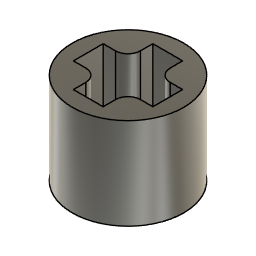
ring (Autodesk Fusion 360 design; units mm, degrees)
Autodesk Fusion 360 part; units mm, degrees
sketch "Sketch1" plane through (0, 0, 0) normal (0, 0, 1) x (1, 0, 0)
  line L0 (-6.1203, 21.0064) -> (-1.3403, 21.0064)
  line L1 (-1.3403, 21.0064) -> (-1.3403, 19.2164)
  line L2 (-1.3403, 19.2164) -> (-6.1203, 19.2164)
  line L3 (-6.1203, 19.2164) -> (-6.1203, 21.0064)
  line L4 (-6.1203, 19.2164) -> (-4.6253, 19.2164)
  line L5 (-4.6253, 19.2164) -> (-2.8353, 19.2164)
  line L6 (-4.6253, 19.2164) -> (-4.6253, 17.7214)
  line L7 (-4.6253, 17.7214) -> (-2.8353, 17.7214)
  line L8 (-2.8353, 17.7214) -> (-2.8353, 17.8)
  line L9 (-2.8353, 17.8) -> (-2.8353, 19.2164)
  line L10 (-4.6253, 19.2164) -> (-4.6253, 21.0064)
  line L11 (-2.8353, 19.2164) -> (-2.8353, 21.0064)
  line L12 (-2.8353, 21.0064) -> (-4.6253, 21.0064)
  line L13 (-4.6253, 21.0064) -> (-4.6253, 22.5014)
  line L14 (-4.6253, 22.5014) -> (-2.8353, 22.5014)
  line L15 (-2.8353, 22.5014) -> (-2.8353, 21.0064)
  circle A0 centre (-5.3728, 18.4689) radius 0.7475
  circle A1 centre (-2.0878, 18.4689) radius 0.7475
  circle A2 centre (-2.0878, 21.7539) radius 0.7475
  circle A3 centre (-5.3728, 21.7539) radius 0.7475
  circle A4 centre (-3.7303, 20.1114) radius 3.35
  dimension "d2" = 4.78
  dimension "d3" = 1.79
  dimension "d4" = 4.78
  dimension "d5" = 1.495
  dimension "d6" = 1.79
  dimension "d7" = 1.495
  dimension "d8" = 1.79
  dimension "d9" = 1.495
  dimension "d10" = 1.79
  dimension "d11" = 1.495
  dimension "d12" = 0.7475
  dimension "d13" = 0.7475
  dimension "d14" = 1.495
  dimension "d15" = 1.495
  dimension "d16" = 1.495
  dimension "d17" = 6.7
  dimension "d18" = 0.895
  dimension "d19" = 0.895
  constraint horizontal L0
  constraint perpendicular L0 L1
  constraint perpendicular L1 L2
  constraint perpendicular L3 L4
  constraint perpendicular L3 L5
  constraint perpendicular L4 L6
  constraint perpendicular L6 L7
  constraint perpendicular L7 L8
  constraint perpendicular L5 L9
  constraint coincident L0 L10.end
  constraint perpendicular L0 L10
  constraint coincident L0 L11.end
  constraint perpendicular L0 L11
  constraint perpendicular L0 L13
  constraint perpendicular L13 L14
  measures "d2" distance of L0.start L0.end
  measures "d3" distance of L0.end L1.end
  measures "d4" distance of L1.end L2.end
  measures "d5" distance of L2.end L4.end
  measures "d6" distance of L4.end L5.end
  measures "d7" distance of L4.end L6.end
  measures "d8" distance of L6.end L7.end
  measures "d9" distance of L10.end L13.end
  measures "d10" distance of L13.end L14.end
  measures "d11" diameter of A0
  measures "d12" distance of L6 A0.centre
  measures "d13" distance of L2 A0.centre
  measures "d14" diameter of A1
  measures "d15" diameter of A3
  measures "d16" diameter of A2
  measures "d17" diameter of A4
  measures "d18" distance of L11 A4.centre
  measures "d19" distance of L12 A4.centre
extrude "Extrude1" add sketch "Sketch1" along normal blind 5.5 contours A3 | A2 | A0 | A1 | A4
equation "d5 = ( ( 4.78 - 1.79 ) / 2 ) * 1 mm"
equation "d12 = ( 1.495 / 2 ) * 1 mm"
equation "d13 = ( 1.495 / 2 ) * 1 mm"
equation "d18 = ( 1.79 / 2 ) * 1 mm"
equation "d19 = ( 1.79 / 2 ) * 1 mm"
